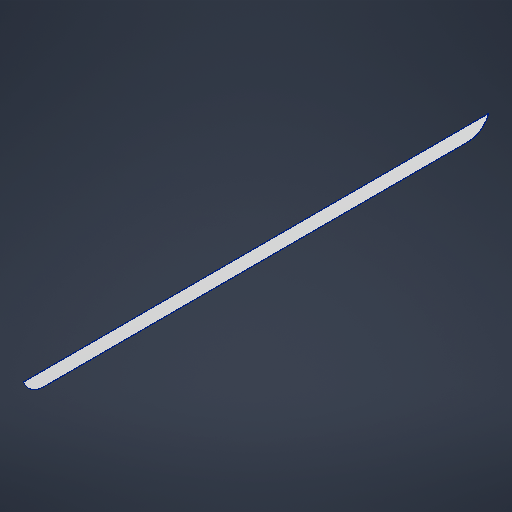
# Autodesk Inventor part: Floor Frame
Saved by Autodesk Inventor 2026 (Build 300175000, 175)
## iProperties
Created: 2025-10-29
Part Number: Floor Frame
Material: Aluminum 6061
Document SubType Name: Sheet Metal
Designer: Brandon Portillo
Density: 2.7 g/cm^3
Sheet Metal Rule: Default_mm
Appearance: Aluminum - Flat
Author: Brandon Portillo
Autodesk Inventor part; units mm, degrees
ref_plane "YZ Plane" through (0, 0, 0) normal (1, 0, 0) x (0, 1, 0)
ref_plane "XZ Plane" through (0, 0, 0) normal (0, 1, 0) x (-1, 0, 0)
ref_plane "XY Plane" through (0, 0, 0) normal (0, 0, 1) x (1, 0, 0)
sketch "Sketch1" plane through (0, 0, 0) normal (1, 0, 0) x (0, 1, 0)
  line L0 (278.0059, 2165.5419) -> (178.0059, 2165.5419)
  line L1 (178.0059, 2165.5419) -> (178.0059, -1084.4581)
  line L2 (178.0059, -1084.4581) -> (278.0059, -1084.4581)
  line L3 (278.0059, -1084.4581) -> (278.0059, 2165.5419)
  dimension "d9" = 100
  dimension "d10" = 3250
  measures "d9" distance of L2.end L1.end
  measures "d10" distance of L1.end L0.end
extrude "Plate1" add sketch "Sketch1" along normal blind 2.3
fillet "Fillet1" radius 150 2 edges at (1.15, 178.0059, 2165.5419) (1.15, 178.0059, -1084.4581)
equation "\"d11\" = Thickness"
equation "\"BendRadius\" = Thickness"
equation "\"BendReliefWidth\" = Thickness"
equation "\"BendReliefDepth\" = 0.5 * Thickness"
equation "\"CornerReliefSize\" = 4 * Thickness"
equation "\"MinimumRemnant\" = 2 * Thickness"
equation "\"TransitionRadius\" = BendRadius"
equation "\"JacobiRadiusSize\" = BendRadius"
equation "\"GapSize\" = Thickness"
equation "\"Thickness\" = 2.3"
body "Solid1"
